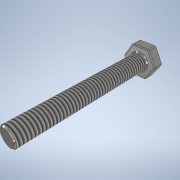
# Autodesk Inventor part: Болт М6х100
Saved by Autodesk Inventor 2021.1 (Build 251245010, 245A)
## iProperties
Created: 2025-12-08
Part Number: Болт М6х100
Material: Типовые
Document SubType Name: Modeling
Designer: Андрей Тарасов
Density: 1 g/cm^3
Appearance: По умолчанию
Author: Андрей Тарасов
Autodesk Inventor part; units mm, degrees
ref_plane "YZ Plane" through (0, 0, 0) normal (1, 0, 0) x (0, 1, 0)
ref_plane "XZ Plane" through (0, 0, 0) normal (0, 1, 0) x (-1, 0, 0)
ref_plane "XY Plane" through (0, 0, 0) normal (0, 0, 1) x (1, 0, 0)
sketch "Эскиз1" plane through (0, 0, 0) normal (0, 0, 1) x (1, 0, 0)
  line L0 (2.8868, 5) -> (5.7735, 0)
  line L1 (5.7735, 0) -> (2.8868, -5)
  line L2 (2.8868, -5) -> (-2.8868, -5)
  line L3 (-2.8868, -5) -> (-5.7735, 0)
  line L4 (-5.7735, 0) -> (-2.8868, 5)
  line L5 (-2.8868, 5) -> (2.8868, 5)
  point P0 (0, 0)
  point P1 (0, 0)
  dimension "d0" = 10
  constraints: 12 end point, 1 coincident, 1 horizontal, 13 other
  measures "d0" distance between parallel lines of L5 L2
extrude "Выдавливание1" add sketch "Эскиз1" along normal blind 4
sketch "Эскиз2" plane through (0, 0, 4) normal (0, 0, 1) x (1, 0, 0)
  circle A0 centre (0, 0) radius 3
  dimension "d3" = 6
  constraints: 1 centre point, 1 coincident
  measures "d3" diameter of A0
extrude "Выдавливание2" add sketch "Эскиз2" along normal blind 45
fillet "Сопряжение1" radius 0.6 6 edges at (2.8868, 5, 2) (-2.8868, 5, 2) (5.7735, 0, 2) (2.8868, -5, 2) (-2.8868, -5, 2) (-5.7735, 0, 2)
chamfer "Фаска1" distance 0.4 angle 45 26 edges at (4.3301, -2.5, 4) (5.6807, 0, 4) (4.3301, 2.5, 4) (2.8403, 4.9196, 4) (0, 5, 4) (-2.8403, 4.9196, 4) (-4.3301, 2.5, 4) (-5.6807, 0, 4) (-4.3301, -2.5, 4) (-2.8403, -4.9196, 4) (0, -5, 4) (2.8403, -4.9196, 4) (4.3301, -2.5, 0) (5.6807, 0, 0) (4.3301, 2.5, 0) (2.8403, 4.9196, 0) (0, 5, 0) (-2.8403, 4.9196, 0) (-4.3301, 2.5, 0) (-5.6807, 0, 0) (-4.3301, -2.5, 0) (-2.8403, -4.9196, 0) (0, -5, 0) (2.8403, -4.9196, 0) (-3, 0, 4) (-3, 0, 49)
thread "Резьба1" size "M6x1" class "6g" standard "ANSI Metric M Profile" full length
